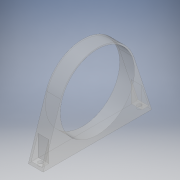
# Autodesk Inventor part: Cap_Mount
Saved by Autodesk Inventor 2016 (Build 200138000, 138)
## iProperties
Created: 2016-05-08
Part Number: Cap_Mount
Material: Polycarbonate, Clear
Document SubType Name: Modeling
Designer: agmle
Density: 1.2 g/cm^3
Appearance: Polycarbonate - Clear
Mass: 82.0248 g
Surface Area: 228.017 cm^2
Volume: 68.354 cm^3
Diameter: 3.934 in
Length: 10.630 in
Cap_Mount_Hole_Diameter: 0.218 in
Cap_Mount_Hole_Spacing: 5.235 in
Cap_Mount_Thickness: 0.782 in
Author: agmle
Autodesk Inventor part; units mm, degrees
ref_plane "YZ Plane" through (0, 0, 0) normal (1, 0, 0) x (0, 1, 0)
ref_plane "XZ Plane" through (0, 0, 0) normal (0, 1, 0) x (-1, 0, 0)
sketch "Sketch1" plane through (0, 0, 0) normal (0, 1, 0) x (-1, 0, 0)
  circle A0 centre (0, 0) radius 49.9618
  arc A1 (16.0964, -49.1656) -> (16.0964, 49.1656) centre (0, 0) ccw
  line L0 (-56.8389, 73.044) -> (-56.8388, -73.0441)
  line L1 (-56.8388, 0) -> (0, 0) construction
  line L2 (-56.8389, 73.044) -> (16.0964, 49.1656)
  line L3 (-56.8388, -73.0441) -> (16.0964, -49.1656)
  line L4 (-51.7335, 42.7443) -> (-51.7334, -42.7443) construction
  dimension "d0" = 99.9236
  dimension "d1" = 103.4669
  dimension "d2" = 146.0881
  dimension "d3" = 5.1054
  constraints: 10 end point, 3 tangent, 2 centre point, 2 coincident, 2 point on circle, 2 vertical, 1 midpoint, 1 perpendicular
  measures "d0" diameter of A0
  measures "d1" diameter of A1
  measures "d2" distance of L0.start L0.end
  measures "d3" distance between parallel lines of L0 L4
extrude "Extrusion1" add sketch "Sketch1" along normal blind 19.8628
ref_plane "Work Plane1" through (53.3591, 0, 73.044) normal (1, 0, 0) x (0, 0, -1)
sketch "Sketch2" plane through (53.3591, 0, 73.044) normal (1, 0, 0) x (0, 0, -1)
  line L0 (146.0881, 0) -> (146.0881, 19.8628) construction
  line L1 (146.0881, 19.8628) -> (122.2096, 19.8628) construction
  line L2 (146.0881, 0) -> (122.2096, 0) construction
  line L3 (23.8785, 19.8628) -> (0, 19.8628) construction
  line L4 (23.8785, 0) -> (0, 0) construction
  line L5 (0, 0) -> (0, 19.8628) construction
  line L6 (23.8785, 0) -> (23.8785, 19.8628) construction
  line L7 (122.2096, 0) -> (122.2096, 19.8628) construction
  line L8 (146.0881, 17.1577) -> (135.763, 17.1577)
  line L9 (135.763, 17.1577) -> (135.763, 2.7051)
  line L10 (135.763, 2.7051) -> (146.0881, 2.7051)
  line L11 (146.0881, 2.7051) -> (146.0881, 17.1577)
  line L12 (0, 17.1577) -> (10.3251, 17.1577)
  line L13 (10.3251, 17.1577) -> (10.3251, 2.7051)
  line L14 (10.3251, 2.7051) -> (0, 2.7051)
  line L15 (0, 2.7051) -> (0, 17.1577)
  point P0 (73.044, 0)
  dimension "d7" = 2.7051
  dimension "d8" = 2.7051
  dimension "d19" = 10.3251
  constraints: 16 end point, 4 parallel, 3 collinear, 2 horizontal, 2 perpendicular, 2 point on line
  measures "d7" distance between parallel lines of L3 L12
  measures "d8" distance between parallel lines of L4 L14
  measures "d19" distance of L9.end L10.end
extrude "Extrusion2" cut sketch "Sketch2" against normal blind 76.2
sketch "Sketch3" plane through (53.3591, 0, 73.044) normal (1, 0, 0) x (0, 0, -1)
  line L0 (139.5285, 9.9314) -> (6.5596, 9.9314) construction
  line L1 (73.044, 0) -> (73.044, 9.9314) construction
  line L2 (135.763, 17.1577) -> (135.763, 2.7051) construction
  line L3 (144.9488, 17.1577) -> (135.763, 17.1577) construction
  line L4 (10.3251, 17.1577) -> (1.1393, 17.1577) construction
  line L5 (144.9488, 17.1577) -> (135.763, 17.1577) construction
  point P0 (73.044, 4.9657)
  point P1 (135.763, 9.9314)
  dimension "Cap_Mount_Hole_Spacing" = 132.969
  constraints: 4 end point, 3 midpoint, 1 perpendicular, 1 point on line, 1 vertical
  measures "Cap_Mount_Hole_Spacing" distance of L0.start L0.end
hole "Hole1" at (53.359, 9.9314, -66.4845) at (53.3591, 9.9314, 66.4845) direction (1, 0, 0) diameter 5.5245 end through all clearance for "Socket Head Cap Screw" size "#10" standard "Ansi Unified Screw Threads"
equation "\"d0\" = Diameter"
equation "\"d8\" = d7"
equation "\"Diameter\" = 99.9236"
body "Solid1"
